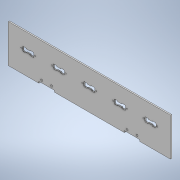
# Autodesk Inventor part: 220207 Front Top
Saved by Autodesk Inventor 2022 (Build 260153000, 153)
## iProperties
Created: 2022-02-07
Part Number: 220207 Front Top
Material: Generic
Document SubType Name: Modeling
Designer: josephinew
Density: 1 g/cm^3
Appearance: Default
Author: josephinew
Autodesk Inventor part; units mm, degrees
ref_plane "YZ Plane" through (0, 0, 0) normal (1, 0, 0) x (0, 1, 0)
ref_plane "XZ Plane" through (0, 0, 0) normal (0, 1, 0) x (-1, 0, 0)
ref_plane "XY Plane" through (0, 0, 0) normal (0, 0, 1) x (1, 0, 0)
sketch "Sketch1" plane through (0, 0, 0) normal (0, 0, 1) x (1, 0, 0)
  line L0 (0, 0) -> (431.8, 0)
  line L1 (431.8, 0) -> (431.8, 101.6)
  line L2 (431.8, 101.6) -> (0, 101.6)
  line L3 (0, 101.6) -> (0, 0)
  dimension "d0" = 431.8
  dimension "d1" = 101.6
  constraints: 8 end point, 2 parallel, 1 horizontal, 1 perpendicular
  measures "d0" distance of L2.end L1.end
  measures "d1" distance of L1.end L0.end
extrude "Extrusion1" add sketch "Sketch1" along normal blind 3.175
sketch "Sketch2" plane through (0, 0, 3.175) normal (0, 0, 1) x (1, 0, 0)
  line L0 (0, 0) -> (38.1, 0)
  circle A0 centre (71.84, 58.27) radius 1.6
  circle A1 centre (34.84, 58.27) radius 1.6
  line L1 (57.5485, 62.47) -> (47.6315, 62.47)
  line L2 (47.6315, 54.07) -> (57.5485, 54.07)
  circle A2 centre (116.12, 58.27) radius 1.6
  circle A3 centre (197.4, 58.27) radius 1.6
  circle A4 centre (278.68, 58.27) radius 1.6
  circle A5 centre (359.96, 58.27) radius 1.6
  arc A6 (47.6315, 62.47) -> (45.79, 64.3115) centre (45.79, 62.47) ccw
  arc A7 (40.34, 64.3115) -> (38.4985, 62.47) centre (40.34, 62.47) ccw
  arc A8 (38.4985, 54.07) -> (40.34, 52.2285) centre (40.34, 54.07) ccw
  arc A9 (45.79, 52.2285) -> (47.6315, 54.07) centre (45.79, 54.07) ccw
  arc A10 (57.5485, 54.07) -> (59.39, 52.2285) centre (59.39, 54.07) ccw
  arc A11 (66.34, 52.2285) -> (68.1815, 54.07) centre (66.34, 54.07) ccw
  arc A12 (68.1815, 62.47) -> (66.34, 64.3115) centre (66.34, 62.47) ccw
  arc A13 (59.39, 64.3115) -> (57.5485, 62.47) centre (59.39, 62.47) ccw
  line L3 (45.79, 64.3115) -> (40.34, 64.3115)
  line L4 (38.4985, 62.47) -> (38.4985, 54.07)
  line L5 (40.34, 52.2285) -> (45.79, 52.2285)
  line L6 (59.39, 52.2285) -> (66.34, 52.2285)
  line L7 (68.1815, 54.07) -> (68.1815, 62.47)
  line L8 (66.34, 64.3115) -> (59.39, 64.3115)
  circle A14 centre (153.12, 58.27) radius 1.6
  line L9 (138.8285, 62.47) -> (128.9115, 62.47)
  line L10 (128.9115, 54.07) -> (138.8285, 54.07)
  arc A15 (128.9115, 62.47) -> (127.07, 64.3115) centre (127.07, 62.47) ccw
  arc A16 (121.62, 64.3115) -> (119.7785, 62.47) centre (121.62, 62.47) ccw
  arc A17 (119.7785, 54.07) -> (121.62, 52.2285) centre (121.62, 54.07) ccw
  arc A18 (127.07, 52.2285) -> (128.9115, 54.07) centre (127.07, 54.07) ccw
  arc A19 (138.8285, 54.07) -> (140.67, 52.2285) centre (140.67, 54.07) ccw
  arc A20 (147.62, 52.2285) -> (149.4615, 54.07) centre (147.62, 54.07) ccw
  arc A21 (149.4615, 62.47) -> (147.62, 64.3115) centre (147.62, 62.47) ccw
  arc A22 (140.67, 64.3115) -> (138.8285, 62.47) centre (140.67, 62.47) ccw
  line L11 (127.07, 64.3115) -> (121.62, 64.3115)
  line L12 (119.7785, 62.47) -> (119.7785, 54.07)
  line L13 (121.62, 52.2285) -> (127.07, 52.2285)
  line L14 (140.67, 52.2285) -> (147.62, 52.2285)
  line L15 (149.4615, 54.07) -> (149.4615, 62.47)
  line L16 (147.62, 64.3115) -> (140.67, 64.3115)
  circle A23 centre (234.4, 58.27) radius 1.6
  line L17 (220.1085, 62.47) -> (210.1915, 62.47)
  line L18 (210.1915, 54.07) -> (220.1085, 54.07)
  arc A24 (210.1915, 62.47) -> (208.35, 64.3115) centre (208.35, 62.47) ccw
  arc A25 (202.9, 64.3115) -> (201.0585, 62.47) centre (202.9, 62.47) ccw
  arc A26 (201.0585, 54.07) -> (202.9, 52.2285) centre (202.9, 54.07) ccw
  arc A27 (208.35, 52.2285) -> (210.1915, 54.07) centre (208.35, 54.07) ccw
  arc A28 (220.1085, 54.07) -> (221.95, 52.2285) centre (221.95, 54.07) ccw
  arc A29 (228.9, 52.2285) -> (230.7415, 54.07) centre (228.9, 54.07) ccw
  arc A30 (230.7415, 62.47) -> (228.9, 64.3115) centre (228.9, 62.47) ccw
  arc A31 (221.95, 64.3115) -> (220.1085, 62.47) centre (221.95, 62.47) ccw
  line L19 (208.35, 64.3115) -> (202.9, 64.3115)
  line L20 (201.0585, 62.47) -> (201.0585, 54.07)
  line L21 (202.9, 52.2285) -> (208.35, 52.2285)
  line L22 (221.95, 52.2285) -> (228.9, 52.2285)
  line L23 (230.7415, 54.07) -> (230.7415, 62.47)
  line L24 (228.9, 64.3115) -> (221.95, 64.3115)
  circle A32 centre (315.68, 58.27) radius 1.6
  line L25 (301.3885, 62.47) -> (291.4715, 62.47)
  line L26 (291.4715, 54.07) -> (301.3885, 54.07)
  arc A33 (291.4715, 62.47) -> (289.63, 64.3115) centre (289.63, 62.47) ccw
  arc A34 (284.18, 64.3115) -> (282.3385, 62.47) centre (284.18, 62.47) ccw
  arc A35 (282.3385, 54.07) -> (284.18, 52.2285) centre (284.18, 54.07) ccw
  arc A36 (289.63, 52.2285) -> (291.4715, 54.07) centre (289.63, 54.07) ccw
  arc A37 (301.3885, 54.07) -> (303.23, 52.2285) centre (303.23, 54.07) ccw
  arc A38 (310.18, 52.2285) -> (312.0215, 54.07) centre (310.18, 54.07) ccw
  arc A39 (312.0215, 62.47) -> (310.18, 64.3115) centre (310.18, 62.47) ccw
  arc A40 (303.23, 64.3115) -> (301.3885, 62.47) centre (303.23, 62.47) ccw
  line L27 (289.63, 64.3115) -> (284.18, 64.3115)
  line L28 (282.3385, 62.47) -> (282.3385, 54.07)
  line L29 (284.18, 52.2285) -> (289.63, 52.2285)
  line L30 (303.23, 52.2285) -> (310.18, 52.2285)
  line L31 (312.0215, 54.07) -> (312.0215, 62.47)
  line L32 (310.18, 64.3115) -> (303.23, 64.3115)
  circle A41 centre (396.96, 58.27) radius 1.6
  line L33 (382.6685, 62.47) -> (372.7515, 62.47)
  line L34 (372.7515, 54.07) -> (382.6685, 54.07)
  arc A42 (372.7515, 62.47) -> (370.91, 64.3115) centre (370.91, 62.47) ccw
  arc A43 (365.46, 64.3115) -> (363.6185, 62.47) centre (365.46, 62.47) ccw
  arc A44 (363.6185, 54.07) -> (365.46, 52.2285) centre (365.46, 54.07) ccw
  arc A45 (370.91, 52.2285) -> (372.7515, 54.07) centre (370.91, 54.07) ccw
  arc A46 (382.6685, 54.07) -> (384.51, 52.2285) centre (384.51, 54.07) ccw
  arc A47 (391.46, 52.2285) -> (393.3015, 54.07) centre (391.46, 54.07) ccw
  arc A48 (393.3015, 62.47) -> (391.46, 64.3115) centre (391.46, 62.47) ccw
  arc A49 (384.51, 64.3115) -> (382.6685, 62.47) centre (384.51, 62.47) ccw
  line L35 (370.91, 64.3115) -> (365.46, 64.3115)
  line L36 (363.6185, 62.47) -> (363.6185, 54.07)
  line L37 (365.46, 52.2285) -> (370.91, 52.2285)
  line L38 (384.51, 52.2285) -> (391.46, 52.2285)
  line L39 (393.3015, 54.07) -> (393.3015, 62.47)
  line L40 (391.46, 64.3115) -> (384.51, 64.3115)
  point P0 (68.09, 58.27)
  point P1 (149.37, 58.27)
  point P2 (230.65, 58.27)
  point P3 (311.93, 58.27)
  point P4 (393.21, 58.27)
  constraints: 82 end point, 80 point on circle, 50 centre point, 20 point on line, 20 tangent, 1 horizontal
extrude "Extrusion2" cut sketch "Sketch2" against normal blind 25.4
sketch "Sketch3" plane through (0, 0, 3.175) normal (0, 0, 1) x (1, 0, 0)
  circle A0 centre (88.9042, 10.795) radius 2.54
  circle A1 centre (115.3202, 10.795) radius 2.54
  circle A2 centre (316.4798, 10.795) radius 2.54
  circle A3 centre (342.8958, 10.795) radius 2.54
  line L0 (0, 101.6) -> (0, 0) projected
  line L1 (0, 0) -> (0, 10.795)
  line L2 (88.9042, 10.795) -> (0, 10.795)
  dimension "d37" = 10.795
  constraints: 4 centre point, 4 end point, 1 horizontal, 1 point on line
  measures "d37" distance of L0.end L1.end
extrude "Extrusion3" cut sketch "Sketch3" against normal blind 3.175
sketch "Sketch4" plane through (0, 0, 3.175) normal (0, 0, 1) x (1, 0, 0)
  circle A0 centre (88.9042, 10.795) radius 2.54 projected
  circle A1 centre (115.3202, 10.795) radius 2.54 projected
  line L0 (102.1122, 0) -> (121.213, 0)
  line L1 (102.1122, 0) -> (83.0114, 0)
  line L2 (83.0114, 0) -> (83.0114, 3.81)
  line L3 (83.0114, 3.81) -> (121.213, 3.81)
  line L4 (121.213, 3.81) -> (121.213, 0)
  line L5 (329.6878, 0) -> (310.587, 0)
  line L6 (329.6878, 0) -> (348.7886, 0)
  line L7 (348.7886, 0) -> (348.7886, 3.81)
  line L8 (348.7886, 3.81) -> (310.587, 3.81)
  line L9 (310.587, 3.81) -> (310.587, 0)
  point P0 (0, 0)
  point P1 (431.8, 0)
  constraints: 20 end point, 2 perpendicular, 1 horizontal
extrude "Extrusion4" cut sketch "Sketch4" against normal blind 3.175 contours L1 L2 L3 L4 L0 | L5 L9 L8 L7 L6
sketch "Sketch8" plane through (0, 0, 3.175) normal (0, 0, 1) x (1, 0, 0)
  line L0 (102.108, 431.8) -> (122.7455, 431.8)
  line L1 (102.108, 431.8) -> (81.4705, 431.8)
  line L2 (81.4705, 431.8) -> (81.4705, 429.26)
  line L3 (121.158, 429.26) -> (83.058, 429.26)
  line L4 (122.7455, 429.26) -> (122.7455, 431.8)
  line L5 (121.158, 429.26) -> (121.158, 431.8)
  line L6 (81.4705, 431.8) -> (81.4705, 427.4312)
  line L7 (81.4705, 427.4312) -> (122.7455, 427.4312)
  line L8 (122.7455, 427.4312) -> (122.7455, 429.26)
  line L9 (83.058, 429.26) -> (83.058, 427.4312)
  line L10 (121.158, 429.26) -> (121.158, 427.4312)
  line L11 (102.108, 431.8) -> (122.7455, 431.8)
  line L12 (102.108, 431.8) -> (81.4705, 431.8)
  line L13 (81.4705, 431.8) -> (81.4705, 429.26)
  line L14 (121.158, 429.26) -> (83.058, 429.26)
  line L15 (122.7455, 429.26) -> (122.7455, 431.8)
  line L16 (121.158, 429.26) -> (121.158, 431.8)
  line L17 (81.4705, 431.8) -> (81.4705, 427.4312)
  line L18 (81.4705, 427.4312) -> (122.7455, 427.4312)
  line L19 (122.7455, 427.4312) -> (122.7455, 429.26)
  line L20 (83.058, 429.26) -> (83.058, 427.4312)
  line L21 (121.158, 429.26) -> (121.158, 427.4312)
  line L22 (102.108, 431.8) -> (122.7455, 431.8)
  line L23 (102.108, 431.8) -> (81.4705, 431.8)
  line L24 (81.4705, 431.8) -> (81.4705, 429.26)
  line L25 (121.158, 429.26) -> (83.058, 429.26)
  line L26 (122.7455, 429.26) -> (122.7455, 431.8)
  line L27 (121.158, 429.26) -> (121.158, 431.8)
  line L28 (81.4705, 431.8) -> (81.4705, 427.4312)
  line L29 (81.4705, 427.4312) -> (122.7455, 427.4312)
  line L30 (122.7455, 427.4312) -> (122.7455, 429.26)
  line L31 (83.058, 429.26) -> (83.058, 427.4312)
  line L32 (121.158, 429.26) -> (121.158, 427.4312)
  line L33 (121.213, 3.81) -> (83.0114, 3.81) projected
  line L34 (102.1122, 3.81) -> (102.1122, 0)
  line L35 (102.1122, 0) -> (122.7497, 0)
  line L36 (121.213, 0) -> (310.587, 0) projected
  line L37 (122.7497, 0) -> (122.7497, 4.3688)
  line L38 (122.7497, 4.3688) -> (81.4747, 4.3688)
  line L39 (81.4747, 4.3688) -> (81.4747, 0)
  line L40 (0, 0) -> (83.0114, 0) projected
  line L41 (83.0114, 0) -> (122.7497, 0)
  line L42 (81.4747, 0) -> (102.1122, 0)
  line L43 (83.0114, 0) -> (83.0114, -1.0374)
  line L44 (310.587, 0) -> (310.587, -4.8026)
  line L45 (329.6878, 3.81) -> (329.6878, 0)
  line L46 (329.6878, 0) -> (350.3253, 0)
  line L47 (350.3253, 0) -> (350.3253, 4.3688)
  line L48 (350.3253, 4.3688) -> (309.0503, 4.3688)
  line L49 (309.0503, 4.3688) -> (309.0503, 0)
  line L50 (310.587, 0) -> (350.3253, 0)
  line L51 (309.0503, 0) -> (329.6878, 0)
  line L52 (310.587, 0) -> (310.587, -1.0374)
  point P0 (83.058, 431.8)
  point P1 (83.058, 431.8)
  point P2 (83.058, 431.8)
  point P3 (102.1122, 0)
  dimension "d55" = 20.6375
  dimension "d56" = 4.3688
  dimension "d57" = 20.6375
  dimension "d58" = 4.3688
  dimension "d59" = 20.6375
  dimension "d60" = 4.3688
  dimension "d61" = 20.6375
  dimension "d62" = 4.3688
  dimension "d63" = 41.275
  dimension "d64" = 20.6375
  dimension "d65" = 4.3688
  dimension "d66" = 41.275
  constraints: 100 end point, 24 perpendicular, 9 vertical, 8 point on line, 3 horizontal, 2 collinear, 1 midpoint
  measures "d55" distance of L0.start L0.end
  measures "d56" distance of L1.end L6.end
  measures "d57" distance of L11.start L11.end
  measures "d58" distance of L12.end L17.end
  measures "d59" distance of L22.start L22.end
  measures "d60" distance of L23.end L29.start
  measures "d61" distance of L34.end L35.end
  measures "d62" distance of L35.end L37.end
  measures "d63" distance of L37.end L38.end
  measures "d64" distance of L51.end L50.end
  measures "d65" distance of L50.end L48.start
  measures "d66" distance of L48.start L48.end
extrude "Extrusion5" cut sketch "Sketch8" against normal blind 25.4 contours L41 L40 L39 L38 L37 L35 | L49 L48 L47 L46 L50 L36
body "Solid1"
